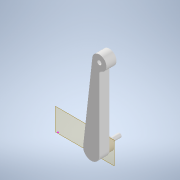
# Autodesk Inventor part: C2
Saved by Autodesk Inventor 2022.2 (Build 262287010, 287A)
## iProperties
Created: 2022-04-11
Part Number: C2
Material: Generic
Document SubType Name: Modeling
Designer: stasi
Density: 1 g/cm^3
Appearance: Default
Author: stasi
Autodesk Inventor part; units mm, degrees
ref_plane "YZ Plane" through (0, 0, 0) normal (1, 0, 0) x (0, 1, 0)
ref_plane "XZ Plane" through (0, 0, 0) normal (0, 1, 0) x (-1, 0, 0)
ref_plane "XY Plane" through (0, 0, 0) normal (0, 0, 1) x (1, 0, 0)
ref_plane "Work Plane1" through (0, 0, 0) normal (0, 0, 1) x (1, 0, 0)
sketch "Sketch1" plane through (0, 0, 0) normal (0, 0, 1) x (1, 0, 0)
  line L0 (0, 0) -> (106.96, 0)
  line L1 (106.96, 0) -> (106.96, 25)
  line L2 (106.96, 25) -> (0, 25)
  line L3 (0, 25) -> (0, 0)
  circle A0 centre (106.96, 25) radius 20
  circle A1 centre (106.96, 25) radius 17.5
  dimension "d0" = 106.96
  dimension "d1" = 25
  dimension "d2" = 40
  dimension "d3" = 35
  constraints: 8 end point, 2 centre point, 2 coincident, 2 parallel, 1 horizontal, 1 perpendicular
  measures "d0" distance of L2.end L1.end
  measures "d1" distance of L1.end L0.end
  measures "d2" diameter of A0
  measures "d3" diameter of A1
extrude "mocowanie we wnece c1" add sketch "Sketch1" against normal blind 15 contours A1 L2 L1 | L1 L2 A1
sketch "Sketch2" plane through (106.96, 25, -15) normal (0, 0, -1) x (-1, 0, 0)
  circle A0 centre (0, 0) radius 5
  point P0 (106.96, -25)
  dimension "d6" = 10
  dimension "d44" = 109.8428
  constraints: 1 centre point
  measures "d6" diameter of A0
  measures "d44" distance of point (106.96, -25) A0.centre
extrude "wal c2" add sketch "Sketch2" along normal blind 30
sketch "Sketch3" plane through (106.96, 25, 0) normal (0, 0, 1) x (1, 0, 0)
  circle A0 centre (0, 0) radius 5 projected
  circle A1 centre (0, 0) radius 20
  line L0 (-106.96, -25) -> (20, -25)
  line L1 (20, 264.9484) -> (-106.96, 264.9484)
  line L2 (-106.96, 264.9484) -> (-106.96, -25)
  circle A2 centre (0, 0) radius 17.5 projected
  line L3 (-106.96, 264.9484) -> (20, 264.9484)
  line L4 (20, 0) -> (-106.96, 0)
  line L5 (-106.96, 0) -> (-106.96, 264.9484)
  circle A3 centre (20, 200) radius 17.5
  circle A4 centre (20, 200) radius 12.5
  line L6 (2.5, 200) -> (-19.7344, 3.2484)
  line L7 (20, 0) -> (20, 200)
  point P0 (20, 182.5)
  dimension "d23" = 35
  dimension "d9" = 40
  dimension "d24" = 25
  dimension "d34" = 6.448
  dimension "d35" = 6.448
  dimension "d36" = 264.9484
  dimension "d37" = 19.9744
  dimension "d38" = 0
  dimension "d39" = 0
  dimension "d40" = 17.3893
  dimension "d41" = 0
  dimension "d42" = 19.3544
  dimension "d43" = 0
  constraints: 16 end point, 3 parallel, 2 centre point, 2 coincident, 2 horizontal, 2 point on circle, 1 perpendicular, 1 tangent, 3 other
  measures "d9" diameter of A1
  measures "d24" diameter of A4
  measures "d34" angle of L6 L7
  measures "d35" angle of L5 L6
  measures "d36" distance between parallel lines of L3 L4
  measures "d37" distance from line of A0.centre L6
  measures "d38" distance from line of L3.end L7
  measures "d39" distance from line of L1.start L7
  measures "d40" distance from line of L7.end L6
  measures "d41" distance from line of point (20, 182.5) L7
  measures "d42" distance from line of point (20, 182.5) L6
  measures "d43" distance from line of L0.end L7
ref_plane "Work Plane2" through (106.96, 25, 0) normal (0, 0, -1) x (-1, 0, 0)
sketch "Sketch5" plane through (106.96, 25, 0) normal (0, 0, -1) x (-1, 0, 0)
  point P0 (106.96, -25)
extrude "trzon c2" add sketch "Sketch3" along normal blind 25 contours L4 A0 | L4 A2 A0 | A0 L4 A2 | A0 L4 | L4 A1 A2 | A2 L4 A1 | A1 L6 A3 L7 | A3 | A4
sketch "Sketch6" plane through (106.96, 25, 0) normal (0, 0, -1) x (-1, 0, 0)
  arc A0 (-2.5, 200) -> (-20, 182.5) centre (-20, 200) ccw projected
  circle A1 centre (-20, 200) radius 12.5
  point P0 (106.96, -25)
  dimension "d27" = 25
  constraints: 1 centre point, 1 coincident
  measures "d27" diameter of A1
extrude "wneka na c3" cut sketch "Sketch6" against normal blind 15
sketch "Sketch7" plane through (126.96, 225, 15) normal (0, 0, -1) x (-1, 0, 0)
  circle A0 centre (0, 0) radius 5
  point P0 (126.96, -225)
  dimension "d30" = 10
  constraints: 1 centre point
  measures "d30" diameter of A0
extrude "dziura na wal c3" cut sketch "Sketch7" against normal blind 10
fillet "Face Fillet2" radius 6 1 edges at (126.96, 207.5, 12.5)
body "Solid1"
